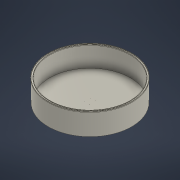
# Autodesk Inventor part: DomeFloorOldMeasurements
Saved by Autodesk Inventor 2022 (Build 260153000, 153)
## iProperties
Created: 2021-05-07
Part Number: DomeFloorOldMeasurements
Material: Generic
Document SubType Name: Modeling
Designer: Mick Veldhuis
Density: 1 g/cm^3
Appearance: Default
Author: Mick Veldhuis
Autodesk Inventor part; units mm, degrees
ref_plane "YZ Plane" through (0, 0, 0) normal (1, 0, 0) x (0, 1, 0)
sketch "Sketch1" plane through (0, 0, 0) normal (0, 1, 0) x (-1, 0, 0)
  circle A0 centre (0, 0) radius 3350
  dimension "d1" = 6700
  constraints: 1 centre point, 1 coincident
  measures "d1" diameter of A0
extrude "Extrusion1" add sketch "Sketch1" along normal blind 100
sketch "Sketch2" plane through (0, 100, 0) normal (0, 1, 0) x (1, 0, 0)
  circle A0 centre (0, 0) radius 3250
  circle A1 centre (0, 0) radius 3350
  constraints: 2 centre point, 2 coincident
extrude "Extrusion2" add sketch "Sketch2" along normal blind 1600
ref_plane "Work Plane1" through (0, 1700, 0) normal (0, 1, 0) x (1, 0, 0)
sketch "Sketch3" plane through (0, 1700, 0) normal (0, 1, 0) x (1, 0, 0)
  circle A0 centre (0, 0) radius 3225
  circle A1 centre (0, 0) radius 3375
  constraints: 2 centre point, 2 coincident
extrude "Extrusion3" add sketch "Sketch3" along normal blind 20
ref_plane "Work Plane2" through (0, 1720, 0) normal (0, 1, 0) x (1, 0, 0)
sketch "Sketch4" plane through (0, 1720, 0) normal (0, 1, 0) x (1, 0, 0)
  circle A0 centre (0, 0) radius 3225
  circle A1 centre (0, 0) radius 3375
  circle A2 centre (0, 0) radius 3250
  circle A3 centre (0, 0) radius 3250 projected
  circle A4 centre (0, 0) radius 3350
  constraints: 4 centre point, 4 coincident
extrude "Extrusion4" add sketch "Sketch4" along normal blind 40
sketch "Sketch5" plane through (0, 100, 0) normal (0, 1, 0) x (1, 0, 0)
  point P0 (180, -230)
  point P1 (-180, -230)
  point P2 (180, 230)
  point P3 (-180, 230)
hole "Hole1" at (180, 100, 230) at (-180, 100, 230) at (180, 100, -230) at (-180, 100, -230) direction (0, -1, 0) diameter 10.106 end through all thread size "M12x1.75" class "6H" standard "ISO Metric profile"
body "Solid1"
